Autodesk Fusion 360 part; units mm, degrees
note: some values were not read from the file. Set by a fixed rule: which face or edge a step refers to.
(part 3 of 3)
sketch "Sketch3" plane through (0, 0, 0) normal (0, -1, 0) x (1, 0, 0)
  line L0 (-40, 18) -> (-40, -18)
  line L1 (-40, -18) -> (40, -18)
  line L2 (40, -18) -> (40, 18)
  line L3 (40, 18) -> (-40, 18)
  line L4 (32.25, -8) -> (-32.25, -8)
  line L5 (-32.25, -8) -> (-32.25, 8)
  line L6 (-32.25, 8) -> (32.25, 8)
  line L7 (32.25, 8) -> (32.25, -8)
  line L8 (-40, 18) -> (40, -18) construction
  line L9 (-37, 15) -> (37, 15) construction
  line L10 (37, 15) -> (37, -15) construction
  line L11 (37, -15) -> (-37, -15) construction
  line L12 (-37, -15) -> (-37, 15) construction
  line L13 (-37, 15) -> (37, -15) construction
  line L14 (37, 15) -> (-37, -15) construction
  circle A0 centre (-37, 15) radius 2
  circle A1 centre (37, 15) radius 2
  circle A2 centre (-37, -15) radius 2
  circle A3 centre (37, -15) radius 2
  dimension "d13" = 74
  dimension "d14" = 4
  dimension "d15" = 4
  dimension "d16" = 4
  dimension "d17" = 4
  constraint coincident L0.start L3.end
  constraint coincident L1.end L2.start
  constraint horizontal L9
  constraint perpendicular L9 L10
  constraint parallel L9 L11
  constraint parallel L10 L12
  constraint coincident L13 origin
  constraint coincident L14 origin
  constraint coincident L9.start L12.end
  constraint coincident L9.end L10.start
  constraint coincident L11.end L12.start
  constraint coincident L10.end L11.start
  measures "d13" distance of L10.end L11.end
  measures "d14" diameter of A0
  measures "d15" diameter of A1
  measures "d16" diameter of A2
  measures "d17" diameter of A3
extrude "Extrude4" cut sketch "Sketch3" against normal blind 1.6 contours A0 | A1 | A2 | A3
fillet "Fillet1" radius 1 4 edges at (32.25, -3.2, 8) (32.25, -3.2, -8) (-32.25, -3.2, 8) (-32.25, -3.2, -8)
fillet "Fillet2" radius 0.5 8 edges at (-31.9571, -6.4, 7.7071) (-32.25, -6.4, 0) (-31.9571, -6.4, -7.7071) (0, -6.4, -8) (31.9571, -6.4, -7.7071) (32.25, -6.4, 0) (31.9571, -6.4, 7.7071) (0, -6.4, 8)
sketch "Sketch4" plane through (0, 0, 0) normal (0, -1, 0) x (1, 0, 0)
  line L0 (31.25, -8) -> (-31.25, -8)
  arc A0 (-32.25, -7) -> (-31.25, -8) centre (-31.25, -7) ccw
  line L1 (-32.25, -7) -> (-32.25, 7)
  arc A1 (-31.25, 8) -> (-32.25, 7) centre (-31.25, 7) ccw
  line L2 (-31.25, 8) -> (31.25, 8)
  arc A2 (32.25, 7) -> (31.25, 8) centre (31.25, 7) ccw
  line L3 (32.25, 7) -> (32.25, -7)
  arc A3 (31.25, -8) -> (32.25, -7) centre (31.25, -7) ccw
  line L4 (-40, 18) -> (-40, -18)
  line L5 (-40, -18) -> (40, -18)
  line L6 (40, -18) -> (40, 18)
  line L7 (40, 18) -> (-40, 18)
  circle A4 centre (37, 15) radius 2
  circle A5 centre (-37, 15) radius 2
  circle A6 centre (37, -15) radius 2
  circle A7 centre (-37, -15) radius 2
  line L8 (-30, 15) -> (-29.5, 15)
  line L9 (-29.5, 15) -> (-29.5, 15.5)
  line L10 (-29.5, 15.5) -> (-30, 15.5)
  line L11 (-30, 15.5) -> (-30, 15)
  dimension "d24" = 0.5
  dimension "d25" = 0.5
  constraint horizontal L8
  constraint vertical L9
  constraint horizontal L10
  constraint vertical L11
  measures "d24" distance of L8.start L8.end
  measures "d25" distance of L8.start L10.end
extrude "Extrude5" add sketch "Sketch4" along normal blind 2 contours L8 L9 L10 L11
fillet "Fillet3" radius 0.5 4 edges at (-29.75, 0, 15.5) (-29.5, 0, 15.25) (-29.75, 0, 15) (-30, 0, 15.25)
fillet "Fillet4" radius 0.1 4 edges at (-29.75, -2, 15.5) (-29.5, -2, 15.25) (-29.75, -2, 15) (-30, -2, 15.25)
pattern_linear "R-Pattern1" count 1 spacing 0 along (0, 0, -1) count 16 spacing 1.6667 along (1, 0, 0) of "Extrude5", "Fillet3", "Fillet4"
fillet "Fillet5" radius 0.5 4 edges at (40, 0.8, 18) (40, 0.8, -18) (-40, 0.8, 18) (-40, 0.8, -18)

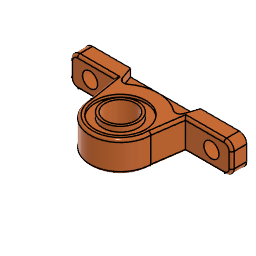
design "PillowBlock"
part number: 2026-09-24-15-42-36-700
Autodesk Fusion 360 part; units mm, degrees
sketch "Sketch1" plane through (0, 0, 0) normal (0, 0, 1) x (1, 0, 0)
  circle A0 centre (0, 0) radius 3
  line L0 (21, 21) -> (-21, 21) construction
  line L1 (-21, 21) -> (-21, -21) construction
  line L2 (-21, -21) -> (21, -21) construction
  line L3 (21, -21) -> (21, 21) construction
  line L4 (21, 21) -> (-21, -21) construction
  line L5 (-21, 21) -> (21, -21) construction
  circle A1 centre (0, 0) radius 6
  line L6 (21, 3) -> (-21, 3)
  line L7 (-21, 3) -> (-21, 9)
  line L8 (-21, 9) -> (21, 9)
  line L9 (21, 9) -> (21, 3)
  line L10 (21, 3) -> (-21, 9) construction
  line L11 (-21, 3) -> (21, 9) construction
  line L12 (0, 6) -> (21, 6)
  line L13 (0, 6) -> (-21, 6)
  line L14 (-6, -0.0008) -> (-6.9902, 6)
  line L15 (6, -0.0004) -> (6.8571, 5.9993)
  line L16 (6.4285, 2.9995) -> (6.8571, 5.9993)
  line L17 (6.4285, 2.9995) -> (6, -0.0004)
  line L18 (6.8571, 5.9993) -> (0, 6)
  point P0 (0, 6)
  dimension "d1" = 6
  dimension "d2" = 42
  dimension "d3" = 42
  dimension "d4" = 12
  dimension "d5" = 162.5
  constraint coincident A0.centre A1.centre
  constraint horizontal L0
  constraint perpendicular L0 L1
  constraint parallel L0 L2
  constraint parallel L1 L3
  constraint coincident L4 A0.centre
  constraint coincident L5 A0.centre
  constraint horizontal L6
  constraint perpendicular L6 L7
  constraint parallel L6 L8
  constraint parallel L7 L9
  constraint coincident L10 P0
  constraint coincident L11 P0
  constraint coincident L3 L6.start
  constraint coincident A1 P0
  constraint coincident P0 L12.start
  constraint midpoint L9 L12.end
  constraint midpoint L7 L13.end
  constraint coincident A1 L14.start
  constraint coincident L13 L14.end
  constraint coincident A1 L15.start
  constraint perpendicular L10 L15
  constraint midpoint L15 L16.start
  measures "d1" diameter of A0
  measures "d2" distance of L1.end L2.end
  measures "d3" distance of L0.end L1.end
  measures "d4" diameter of A1
  measures "d5" angle of L14 L15
extrude "Extrude1" add sketch "Sketch1" along normal blind 12 contours A1 L6 | A1 L6 | A1 L6 L15 L17 | A1 L6 L13 L14 | A1 L6 L14 | L7 L8 L9 L12 L13 L18
sketch "Sketch2" plane through (0, 0, 12) normal (0, 0, 1) x (-1, 0, 0)
  circle A0 centre (0, 0) radius 3
  arc A1 (6, 0.0008) -> (-6, 0.0004) centre (0, 0) ccw
  line L0 (-6, 0.0004) -> (-6.4286, -3)
  line L1 (-6.4286, -3) -> (-5.1962, -3)
  arc A2 (-5.1962, -3) -> (0, -6) centre (0, 0) ccw
  line L2 (0, -6) -> (-21, -6)
  line L3 (-21, -6) -> (-21, -9)
  line L4 (-21, -9) -> (21, -9)
  line L5 (21, -9) -> (21, -6)
  line L6 (21, -6) -> (6.9902, -6)
  line L7 (6.9902, -6) -> (6, 0.0008)
  line L8 (-6.2143, -1.4998) -> (-6.8572, -6)
  constraint midpoint L0 L8.start
  constraint coincident L2 L8.end
  constraint parallel L0 L8
extrude "Extrude2" add sketch "Sketch2" against normal blind 12 contours L1 A2 L2 L8
sketch "Sketch3" plane through (0, 0, 0) normal (0, 0, -1) x (1, 0, 0)
  circle A0 centre (0, 0) radius 3
  arc A1 (6, 0.0004) -> (-6, 0.0008) centre (0, 0) ccw
  line L0 (-6, 0.0008) -> (-6.9902, -6)
  line L1 (-6.9902, -6) -> (-21, -6)
  line L2 (-21, -6) -> (-21, -9)
  line L3 (-21, -9) -> (21, -9)
  line L4 (21, -9) -> (21, -6)
  line L5 (21, -6) -> (6.8572, -6)
  line L6 (6.8572, -6) -> (6, 0.0004)
  circle A2 centre (0, 0) radius 5
  dimension "d10" = 10
  constraint coincident A0.centre A1.centre
  measures "d10" diameter of A2
extrude "Extrude3" cut sketch "Sketch3" against normal blind 0.5 contours A2
sketch "Sketch4" plane through (0, 0, 0) normal (0, 0, -1) x (1, 0, 0)
  circle A0 centre (0, 0) radius 5
  arc A1 (6, 0.0004) -> (-6, 0.0008) centre (0, 0) ccw
  line L0 (-6, 0.0008) -> (-6.9902, -6)
  line L1 (-6.9902, -6) -> (-21, -6)
  line L2 (-21, -6) -> (-21, -9)
  line L3 (-21, -9) -> (21, -9)
  line L4 (21, -9) -> (21, -6)
  line L5 (21, -6) -> (6.8572, -6)
  line L6 (6.8572, -6) -> (6, 0.0004)
  line L7 (-6.9902, -9) -> (-6.9902, -6)
  line L8 (6.8572, -6) -> (6.8572, -9)
  line L9 (-4.8731, -4.9988) -> (4.8504, -4.9988)
  circle A2 centre (0, 0) radius 7.4924
  line L10 (5.8031, -5.6949) -> (6.8572, -9)
  line L11 (-5.8163, -5.6666) -> (-6.9902, -9)
  arc A3 (-4.8731, -4.9988) -> (-5.8163, -5.6666) centre (-4.8731, -5.9988) ccw
  arc A4 (5.8031, -5.6949) -> (4.8504, -4.9988) centre (4.8504, -5.9988) ccw
  dimension "d13" = 1
  constraint coincident L3 L7.start
  constraint coincident L0.end L1.start
  constraint perpendicular L1 L7
  constraint coincident L5.end L6.start
  constraint coincident L3 L8.end
  constraint perpendicular L3 L8
  constraint perpendicular L7 L9
  constraint coincident A0.centre A1.centre
  constraint tangent L11 A3
  constraint tangent L9 A3
  constraint tangent L10 A4
  constraint tangent L9 A4
  constraint equal A3 A4
  measures "d13" radius of A3
extrude "Extrude4" cut sketch "Sketch4" against normal blind 12 contours L3 A2 L10 L11 A3 A4
fillet "Fillet1" radius 1 2 edges at (-5.4267, 5.166, 6) (5.4178, 5.1753, 6)
sketch "Sketch5" plane through (0, 9, 0) normal (0, 1, 0) x (-1, 0, 0)
  line L0 (6.9902, 12) -> (6.9902, 0)
  line L1 (6.9902, 0) -> (21, 0)
  line L2 (21, 0) -> (21, 12)
  line L3 (21, 12) -> (6.9902, 12)
  line L4 (-21, 12) -> (21, 0) construction
  line L5 (21, 3) -> (-21, 3)
  line L6 (-21, 3) -> (-21, 9)
  line L7 (-21, 9) -> (21, 9)
  line L8 (21, 9) -> (21, 3)
  line L9 (21, 3) -> (-21, 9) construction
  line L10 (-21, 3) -> (21, 9) construction
  point P0 (0, 6)
  dimension "d18" = 6
  constraint coincident L1.end L2.start
  constraint horizontal L5
  constraint perpendicular L5 L6
  constraint parallel L5 L7
  constraint parallel L6 L8
  constraint coincident L9 P0
  constraint coincident L10 P0
  constraint midpoint L4 P0
  measures "d18" distance of L5.end L6.end
extrude "Extrude5" add sketch "Sketch5" against normal blind 3 contours L0 L2 L5 L7 L8 | L0 L5 L6 L7
sketch "Sketch6" plane through (0, 0, 12) normal (0, 0, 1) x (-1, 0, 0)
  line L0 (-6.8572, -9) -> (-6.0551, -6.4849)
  arc A0 (-4.5015, -5.9894) -> (-6.0551, -6.4849) centre (-5.1024, -6.7888) ccw
  arc A1 (-4.5015, -5.9894) -> (4.5356, -5.9636) centre (0, 0) ccw
  arc A2 (6.0842, -6.4274) -> (4.5356, -5.9636) centre (5.141, -6.7596) ccw
  line L1 (6.0842, -6.4274) -> (6.9902, -9)
  line L2 (6.9902, -9) -> (21, -9)
  line L3 (21, -9) -> (21, -6)
  line L4 (21, -6) -> (6.9902, -6)
  line L5 (6.9902, -6) -> (6, 0.0008)
  arc A3 (6, 0.0008) -> (-6, 0.0004) centre (0, 0) ccw
  line L6 (-6, 0.0004) -> (-6.8572, -6)
  line L7 (-6.8572, -6) -> (-21, -6)
  line L8 (-21, -6) -> (-21, -9)
  line L9 (-21, -9) -> (-6.8572, -9)
  circle A4 centre (0, 0) radius 3
  circle A5 centre (0, 0) radius 5
  dimension "d21" = 10
  constraint concentric A1 A5
  measures "d21" diameter of A5
extrude "Extrude6" cut sketch "Sketch6" against normal blind 0.5 contours A5
sketch "Sketch7" plane through (0, 0, 0.5) normal (0, 0, -1) x (1, 0, 0)
  circle A0 centre (0, 0) radius 3
  circle A1 centre (0, 0) radius 5
  circle A2 centre (0, 0) radius 3.5
  dimension "d24" = 7
  constraint coincident A0.centre A1.centre
  measures "d24" diameter of A2
extrude "Extrude7" add sketch "Sketch7" along normal blind 1 contours A2
extrude "Extrude8" add 1 faces at (3.3203, 0.1739, -0.5) along direction (0, 0, 1) blind 13
extrude "Extrude9" cut 1 faces at (11.5714, 6.9998, 12) along direction (0, 0, -1) blind 6
extrude "Extrude10" cut 1 faces at (-4.4814, 0.2484, 11.5) along direction (0, 0, -1) blind 6
extrude "Extrude11" cut 1 faces at (3.3203, 0.1739, 12.5) along direction (0, 0, -1) blind 6
extrude "Extrude12" cut 1 faces at (0.1337, 8.4911, 9) along direction (0, 0, -1) blind 6
sketch "Sketch8" plane through (0, 9, 0) normal (0, 1, 0) x (-1, 0, 0)
  line L0 (-6.8572, 0) -> (-6.8572, 6)
  line L1 (-6.8572, 6) -> (-21, 6)
  line L2 (-21, 6) -> (-21, 0)
  line L3 (-21, 0) -> (-6.8572, 0)
  line L4 (21, 0) -> (-21, 6) construction
  line L5 (-21, 4.5) -> (21, 4.5)
  line L6 (21, 4.5) -> (21, 1.5)
  line L7 (21, 1.5) -> (-21, 1.5)
  line L8 (-21, 1.5) -> (-21, 4.5)
  line L9 (-21, 4.5) -> (21, 1.5) construction
  line L10 (21, 4.5) -> (-21, 1.5) construction
  point P0 (0, 3)
  dimension "d37" = 3
  constraint coincident L1.end L2.start
  constraint horizontal L5
  constraint perpendicular L5 L6
  constraint parallel L5 L7
  constraint parallel L6 L8
  constraint coincident L9 P0
  constraint coincident L10 P0
  constraint midpoint L4 P0
  measures "d37" distance of L5.end L6.end
extrude "Extrude13" add sketch "Sketch8" against normal blind 3 contours L0 L2 L5 L7 L8 | L0 L5 L6 L7
extrude "Extrude14" cut 4 faces at (-21, 7, 0.5) (-21, 8, 5.5) (-21, 7, 2) (-21, 7, 3.5) along direction (1, 0, 0) blind 5
extrude "Extrude15" cut 4 faces at (21, 7, 2.5) (21, 8, 0.5) (21, 8, 3.5) (21, 7, 5.5) along direction (-1, 0, 0) blind 5
fillet "Fillet2" radius 1.5 4 edges at (-16, 7.5, 6) (-16, 7.5, 0) (16, 7.5, 0) (16, 7.5, 6)
sketch "Sketch9" plane through (0, 6, 0) normal (0, -1, 0) x (1, 0, 0)
  arc A0 (16, 4.5) -> (14.5, 6) centre (14.5, 4.5) ccw
  line L0 (14.5, 6) -> (6.8572, 6)
  line L1 (6.8572, 6) -> (6.8572, 0)
  line L2 (6.8572, 0) -> (14.5, 0)
  arc A1 (14.5, 0) -> (16, 1.5) centre (14.5, 1.5) ccw
  line L3 (16, 1.5) -> (16, 4.5)
  line L4 (16, 3) -> (12, 3) construction
  circle A2 centre (12, 3) radius 1.5
  dimension "d46" = 4
  dimension "d47" = 3
  constraint midpoint L3 L4.start
  constraint perpendicular L3 L4
  constraint coincident L4.end A2.centre
  measures "d46" distance of L4.start L4.end
  measures "d47" diameter of A2
extrude "Extrude16" cut sketch "Sketch9" against normal blind 3 contours A2
sketch "Sketch10" plane through (0, 6, 0) normal (0, -1, 0) x (1, 0, 0)
  arc A0 (-16, 1.5) -> (-14.5, 0) centre (-14.5, 1.5) ccw
  line L0 (-14.5, 0) -> (-6.9902, 0)
  line L1 (-6.9902, 0) -> (-6.9902, 6)
  line L2 (-6.9902, 6) -> (-14.5, 6)
  arc A1 (-14.5, 6) -> (-16, 4.5) centre (-14.5, 4.5) ccw
  line L3 (-16, 4.5) -> (-16, 1.5)
  line L4 (-16, 3) -> (-12, 3) construction
  circle A2 centre (-12, 3) radius 1.5
  dimension "d50" = 4
  dimension "d51" = 3
  constraint midpoint L3 L4.start
  constraint perpendicular L3 L4
  constraint coincident L4.end A2.centre
  measures "d50" distance of L4.start L4.end
  measures "d51" diameter of A2
extrude "Extrude17" cut sketch "Sketch10" against normal blind 3 contours A2
fillet "Fillet3" radius 0.5 16 edges at (0.0002, -6, 6) (-6.4951, 2.9996, 6) (6.4286, 2.9998, 6) (10.6786, 6, 0) (15.5607, 6, 0.4393) (16, 6, 3) (15.5607, 6, 5.5607) (10.6786, 6, 6) (-10.7451, 6, 6) (-15.5607, 6, 5.5607) (-16, 6, 3) (-15.5607, 6, 0.4393) (-10.7451, 6, 0) (-6.4951, 2.9996, 0) (0.0002, -6, 0) (6.4286, 2.9998, 0)

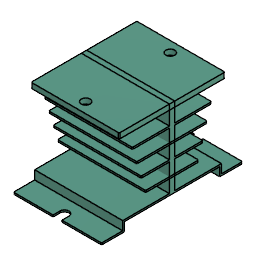
design "SSR_Heatsink"
part number: 2026-09-24-14-46-01-053
Autodesk Fusion 360 part; units mm, degrees
sketch "Sketch1" plane through (0, 0, 0) normal (0, 0, 1) x (1, 0, 0)
  line L0 (-25, 40) -> (25, 40) construction
  line L1 (25, 40) -> (25, -40) construction
  line L2 (25, -40) -> (-25, -40) construction
  line L3 (-25, -40) -> (-25, 40) construction
  line L4 (-25, 40) -> (25, -40) construction
  line L5 (25, 40) -> (-25, -40) construction
  line L6 (-25, 40) -> (25, 40)
  line L7 (25, 40) -> (25, 28)
  line L8 (25, 28) -> (-25, 28)
  line L9 (-25, 28) -> (-25, 40)
  line L10 (-25, -40) -> (25, -40)
  line L11 (25, -40) -> (25, -28)
  line L12 (25, -28) -> (-25, -28)
  line L13 (-25, -28) -> (-25, -40)
  dimension "d1" = 50
  dimension "d2" = 80
  dimension "d3" = 50
  dimension "d4" = 12
  dimension "d5" = 12
  constraint horizontal L0
  constraint perpendicular L0 L1
  constraint parallel L0 L2
  constraint parallel L1 L3
  constraint coincident L4 origin
  constraint coincident L5 origin
  constraint horizontal L6
  constraint vertical L7
  constraint horizontal L8
  constraint vertical L9
  constraint horizontal L10
  constraint vertical L11
  constraint horizontal L12
  constraint vertical L13
  measures "d1" distance of L1.end L2.end
  measures "d2" distance of L0.end L1.end
  measures "d3" distance of L0.start L0.end
  measures "d4" distance of L0.start L8.end
  measures "d5" distance of L2.end L12.end
extrude "Extrude1" add sketch "Sketch1" along normal blind 1 makes body 1 at (-8.3333, 36, 0) makes body 2 at (-8.3333, -32, 0)
sketch "Sketch2" plane through (0, 0, 0) normal (0, 0, 1) x (1, 0, 0)
  line L0 (-25, 40) -> (25, 40)
  line L1 (25, 40) -> (25, -40)
  line L2 (25, -40) -> (-25, -40)
  line L3 (-25, -40) -> (-25, 40)
  line L4 (-25, 40) -> (25, -40) construction
  line L5 (25, 40) -> (-25, -40) construction
  line L6 (-25, 28) -> (25, 28)
  line L7 (25, 28) -> (25, 27)
  line L8 (25, 27) -> (-25, 27)
  line L9 (-25, 27) -> (-25, 28)
  line L10 (-25, -28) -> (25, -28)
  line L11 (25, -28) -> (25, -27)
  line L12 (25, -27) -> (-25, -27)
  line L13 (-25, -27) -> (-25, -28)
  dimension "d8" = 1
  dimension "d9" = 1
  constraint horizontal L0
  constraint perpendicular L0 L1
  constraint parallel L0 L2
  constraint parallel L1 L3
  constraint coincident L4 origin
  constraint coincident L5 origin
  constraint horizontal L6
  constraint vertical L7
  constraint horizontal L8
  constraint vertical L9
  constraint coincident L3 L6.start
  constraint horizontal L10
  constraint vertical L11
  constraint horizontal L12
  constraint vertical L13
  constraint coincident L3 L10.start
  measures "d8" distance of L6.start L8.end
  measures "d9" distance of L10.start L12.end
extrude "Extrude2" add sketch "Sketch2" along normal blind 5 contours L1 L3 L6 L7 L8 L9 | L1 L3 L10 L11 L12 L13 bodies 1 2
ref_plane "WorkPlane1" through (0, -27.5, 5) normal (0, 0, 1) x (1, 0, 0)
sketch "Sketch3" plane through (0, 0, 5) normal (0, 0, 1) x (1, 0, 0)
  line L0 (-25, 28) -> (25, 28)
  line L1 (25, 28) -> (25, -28)
  line L2 (25, -28) -> (-25, -28)
  line L3 (-25, -28) -> (-25, 28)
  line L4 (-25, 28) -> (25, -28) construction
  line L5 (25, 28) -> (-25, -28) construction
  constraint horizontal L0
  constraint perpendicular L0 L1
  constraint parallel L0 L2
  constraint parallel L1 L3
  constraint coincident L4 origin
  constraint coincident L5 origin
extrude "Extrude3" add sketch "Sketch3" along normal blind 1 bodies 1 2
sketch "Sketch4" plane through (0, 0, 6) normal (0, 0, 1) x (-1, 0, 0)
  line L0 (25, 28) -> (-25, 28)
  line L1 (-25, 28) -> (-25, -28)
  line L2 (-25, -28) -> (25, -28)
  line L3 (25, -28) -> (25, 28)
  line L4 (-25, 15) -> (25, 15)
  line L5 (25, 15) -> (25, -15)
  line L6 (25, -15) -> (-25, -15)
  line L7 (-25, -15) -> (-25, 15)
  line L8 (-25, 15) -> (25, -15) construction
  line L9 (25, 15) -> (-25, -15) construction
  line L10 (25, 1.5) -> (-25, 1.5)
  line L11 (-25, 1.5) -> (-25, -1.5)
  line L12 (-25, -1.5) -> (25, -1.5)
  line L13 (25, -1.5) -> (25, 1.5)
  line L14 (25, 1.5) -> (-25, -1.5) construction
  line L15 (-25, 1.5) -> (25, -1.5) construction
  dimension "d15" = 30
  dimension "d16" = 3
  constraint horizontal L4
  constraint perpendicular L4 L5
  constraint parallel L4 L6
  constraint parallel L5 L7
  constraint coincident L8 origin
  constraint coincident L9 origin
  constraint horizontal L10
  constraint perpendicular L10 L11
  constraint parallel L10 L12
  constraint parallel L11 L13
  constraint coincident L14 origin
  constraint coincident L15 origin
  measures "d15" distance of L4.end L5.end
  measures "d16" distance of L10.end L11.end
extrude "Extrude4" add sketch "Sketch4" along normal blind 44 contours L1 L3 L5 L7 L10 L11 L12 L13 bodies 1
ref_plane "WorkPlane2" through (0, 14.75, 13.3) normal (0, 0, 1) x (1, 0, 0)
sketch "Sketch5" plane through (0, 0, 13.3) normal (0, 0, 1) x (1, 0, 0)
  line L0 (25, -15) -> (-25, -15)
  line L1 (-25, -15) -> (-25, 15)
  line L2 (-25, 15) -> (25, 15)
  line L3 (25, 15) -> (25, -15)
  line L4 (25, -15) -> (-25, 15) construction
  line L5 (-25, -15) -> (25, 15) construction
  constraint horizontal L0
  constraint perpendicular L0 L1
  constraint parallel L0 L2
  constraint parallel L1 L3
  constraint coincident L4 origin
  constraint coincident L5 origin
extrude "Extrude5" add sketch "Sketch5" along normal blind 1 separate body makes body 3
ref_plane "WorkPlane3" through (0, 0, 21.6) normal (0, 0, 1) x (1, 0, 0)
sketch "Sketch6" plane through (0, 0, 21.6) normal (0, 0, 1) x (1, 0, 0)
  line L0 (25, -17.5) -> (-25, -17.5)
  line L1 (-25, -17.5) -> (-25, 17.5)
  line L2 (-25, 17.5) -> (25, 17.5)
  line L3 (25, 17.5) -> (25, -17.5)
  line L4 (25, -17.5) -> (-25, 17.5) construction
  line L5 (-25, -17.5) -> (25, 17.5) construction
  dimension "d23" = 35
  constraint horizontal L0
  constraint perpendicular L0 L1
  constraint parallel L0 L2
  constraint parallel L1 L3
  constraint coincident L4 origin
  constraint coincident L5 origin
  measures "d23" distance of L0.end L1.end
extrude "Extrude6" add sketch "Sketch6" along normal blind 1 bodies 1
ref_plane "WorkPlane4" through (0, 9.5, 29.9) normal (0, 0, 1) x (1, 0, 0)
sketch "Sketch7" plane through (0, 0, 29.9) normal (0, 0, 1) x (1, 0, 0)
  line L0 (25, -20) -> (-25, -20)
  line L1 (-25, -20) -> (-25, 20)
  line L2 (-25, 20) -> (25, 20)
  line L3 (25, 20) -> (25, -20)
  line L4 (25, -20) -> (-25, 20) construction
  line L5 (-25, -20) -> (25, 20) construction
  dimension "d27" = 50
  dimension "d28" = 40
  constraint horizontal L0
  constraint perpendicular L0 L1
  constraint parallel L0 L2
  constraint parallel L1 L3
  constraint coincident L4 origin
  constraint coincident L5 origin
  measures "d27" distance of L1.end L2.end
  measures "d28" distance of L0.end L1.end
extrude "Extrude7" add sketch "Sketch7" along normal blind 1 separate body makes body 4
ref_plane "WorkPlane5" through (0, 0, 38.2) normal (0, 0, 1) x (1, 0, 0)
sketch "Sketch8" plane through (0, 0, 38.2) normal (0, 0, 1) x (1, 0, 0)
  line L0 (25, -22.5) -> (-25, -22.5)
  line L1 (-25, -22.5) -> (-25, 22.5)
  line L2 (-25, 22.5) -> (25, 22.5)
  line L3 (25, 22.5) -> (25, -22.5)
  line L4 (25, -22.5) -> (-25, 22.5) construction
  line L5 (-25, -22.5) -> (25, 22.5) construction
  dimension "d32" = 45
  constraint horizontal L0
  constraint perpendicular L0 L1
  constraint parallel L0 L2
  constraint parallel L1 L3
  constraint coincident L4 origin
  constraint coincident L5 origin
  measures "d32" distance of L0.end L1.end
extrude "Extrude8" add sketch "Sketch8" along normal blind 1 bodies 1
ref_plane "WorkPlane6" through (0, 0, 50) normal (0, 0, 1) x (1, 0, 0)
sketch "Sketch9" plane through (0, 0, 50) normal (0, 0, 1) x (1, 0, 0)
  line L0 (25, -30) -> (-25, -30)
  line L1 (-25, -30) -> (-25, 30)
  line L2 (-25, 30) -> (25, 30)
  line L3 (25, 30) -> (25, -30)
  line L4 (25, -30) -> (-25, 30) construction
  line L5 (-25, -30) -> (25, 30) construction
  dimension "d36" = 50
  dimension "d37" = 60
  constraint horizontal L0
  constraint perpendicular L0 L1
  constraint parallel L0 L2
  constraint parallel L1 L3
  constraint coincident L4 origin
  constraint coincident L5 origin
  measures "d36" distance of L1.end L2.end
  measures "d37" distance of L0.end L1.end
extrude "Extrude9" add sketch "Sketch9" against normal blind 3 separate body makes body 5
sketch "Sketch10" plane through (0, 0, 50) normal (0, 0, 1) x (-1, 0, 0)
  line L0 (-25, -30) -> (25, -30)
  line L1 (25, -30) -> (25, 30)
  line L2 (25, 30) -> (-25, 30)
  line L3 (-25, 30) -> (-25, -30)
  line L4 (-24, 24) -> (24, 24) construction
  line L5 (24, 24) -> (24, -24) construction
  line L6 (24, -24) -> (-24, -24) construction
  line L7 (-24, -24) -> (-24, 24) construction
  line L8 (-24, 24) -> (24, -24) construction
  line L9 (24, 24) -> (-24, -24) construction
  circle A0 centre (0, 24) radius 2.5
  circle A1 centre (0, -24) radius 2.5
  dimension "d40" = 48
  dimension "d41" = 48
  dimension "d42" = 5
  dimension "d43" = 5
  constraint horizontal L4
  constraint perpendicular L4 L5
  constraint parallel L4 L6
  constraint parallel L5 L7
  constraint coincident L8 origin
  constraint coincident L9 origin
  constraint midpoint L4 A0.centre
  constraint midpoint L6 A1.centre
  measures "d40" distance of L5.end L6.end
  measures "d41" distance of L4.end L5.end
  measures "d42" diameter of A0
  measures "d43" diameter of A1
extrude "Extrude10" cut sketch "Sketch10" against normal blind 3 contours A0 | A1 bodies 5
sketch "Sketch11" plane through (0, 0, 1) normal (0, 0, 1) x (-1, 0, 0)
  line L0 (25, -28) -> (-25, -28)
  line L1 (-25, -28) -> (-25, -40)
  line L2 (-25, -40) -> (25, -40)
  line L3 (25, -40) -> (25, -28)
  line L4 (2.5, -44) -> (2.5, -36)
  arc A0 (2.5, -36) -> (-2.5, -36) centre (0, -36) ccw
  line L5 (-2.5, -36) -> (-2.5, -44)
  arc A1 (-2.5, -44) -> (2.5, -44) centre (0, -44) ccw
  line L6 (0, -44) -> (0, -36) construction
  point P0 (0, -40)
  dimension "d46" = 5
  constraint tangent L4 A0
  constraint tangent A0 L5
  constraint parallel L4 L5
  constraint tangent L5 A1
  constraint tangent L4 A1
  constraint perpendicular L2 L6
  constraint midpoint L2 P0
  constraint midpoint L6 P0
  measures "d46" diameter of A0
extrude "Extrude11" cut sketch "Sketch11" against normal blind 1 contours L2 L4 A0 L5 bodies 1
sketch "Sketch12" plane through (0, 0, 1) normal (0, 0, 1) x (-1, 0, 0)
  line L0 (25, 28) -> (25, 40)
  line L1 (25, 40) -> (-25, 40)
  line L2 (-25, 40) -> (-25, 28)
  line L3 (-25, 28) -> (25, 28)
  line L4 (-2.5, 44) -> (-2.5, 36)
  arc A0 (-2.5, 36) -> (2.5, 36) centre (0, 36) ccw
  line L5 (2.5, 36) -> (2.5, 44)
  arc A1 (2.5, 44) -> (-2.5, 44) centre (0, 44) ccw
  line L6 (0, 44) -> (0, 36) construction
  point P0 (0, 40)
  dimension "d49" = 5
  constraint tangent L4 A0
  constraint tangent A0 L5
  constraint parallel L4 L5
  constraint tangent L5 A1
  constraint tangent L4 A1
  constraint perpendicular L1 L6
  constraint midpoint L1 P0
  constraint midpoint L6 P0
  measures "d49" diameter of A0
extrude "Extrude12" cut sketch "Sketch12" against normal blind 1 contours L1 L4 A0 L5 bodies 1
fillet "Fillet1" radius 0.5 23 edges at (25, -22.5, 38.7) (25, -17.5, 22.1) (25, -40, 0.5) (-25, -40, 0.5) (25, 40, 0.5) (25, 17.5, 22.1) (25, 22.5, 38.7) (-25, 40, 0.5) (-25, 17.5, 22.1) (-25, -22.5, 38.7) (-25, -17.5, 22.1) (25, -15, 13.8) (25, 15, 13.8) (-25, 15, 13.8) (-25, -15, 13.8) (25, -20, 30.4) (25, 20, 30.4) (-25, 20, 30.4) (-25, -20, 30.4) (25, -30, 48.5) (25, 30, 48.5) (-25, 30, 48.5) (-25, -30, 48.5) on bodies 1 3 4 5

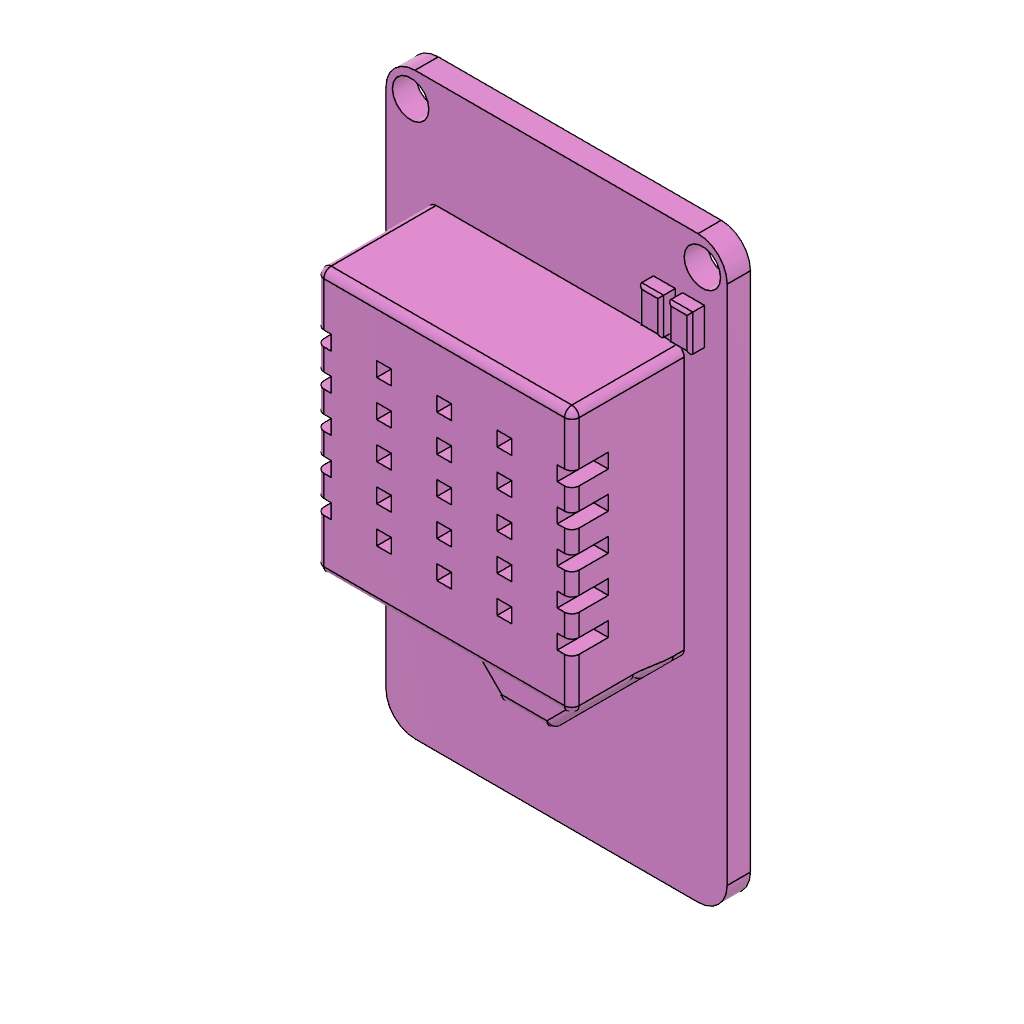
design "DHT22"
part number: 2026-09-25-09-54-51-033
Autodesk Fusion 360 part; units mm, degrees
sketch "Sketch1" plane through (0, 0, 0) normal (0, 0, 1) x (1, 0, 0)
  line L0 (-11.7, 19.85) -> (11.7, 19.85)
  line L1 (11.7, 19.85) -> (11.7, -19.85)
  line L2 (11.7, -19.85) -> (-11.7, -19.85)
  line L3 (-11.7, -19.85) -> (-11.7, 19.85)
  line L4 (-11.7, 19.85) -> (11.7, -19.85) construction
  line L5 (11.7, 19.85) -> (-11.7, -19.85) construction
  dimension "d1" = 23.4
  dimension "d2" = 39.7
  constraint horizontal L0
  constraint perpendicular L0 L1
  constraint parallel L0 L2
  constraint parallel L1 L3
  constraint coincident L4 origin
  constraint coincident L5 origin
  measures "d1" distance of L1.end L2.end
  measures "d2" distance of L0.end L1.end
extrude "Extrude1" add sketch "Sketch1" along normal blind 1.6
sketch "Sketch2" plane through (0, 0, 1.6) normal (0, 0, 1) x (1, 0, 0)
  line L0 (-11.7, -19.85) -> (11.7, -19.85)
  line L1 (11.7, -19.85) -> (11.7, 19.85)
  line L2 (11.7, 19.85) -> (-11.7, 19.85)
  line L3 (-11.7, 19.85) -> (-11.7, -19.85)
  line L4 (-8.75, 12.55) -> (8.75, 12.55)
  line L5 (8.75, 12.55) -> (8.75, -12.55)
  line L6 (8.75, -12.55) -> (-8.75, -12.55)
  line L7 (-8.75, -12.55) -> (-8.75, 12.55)
  line L8 (-8.75, 12.55) -> (8.75, -12.55) construction
  line L9 (8.75, 12.55) -> (-8.75, -12.55) construction
  dimension "d5" = 17.5
  dimension "d6" = 25.1
  constraint horizontal L4
  constraint perpendicular L4 L5
  constraint parallel L4 L6
  constraint parallel L5 L7
  constraint coincident L8 origin
  constraint coincident L9 origin
  measures "d5" distance of L5.end L6.end
  measures "d6" distance of L4.end L5.end
extrude "Extrude2" add sketch "Sketch2" along normal blind 7.7 contours L4 L5 L6 L7
sketch "Sketch3" plane through (0, 0, 9.3) normal (0, 0, 1) x (1, 0, 0)
  line L0 (-8.75, -12.55) -> (8.75, -12.55)
  line L1 (8.75, -12.55) -> (8.75, 12.55)
  line L2 (8.75, 12.55) -> (-8.75, 12.55)
  line L3 (-8.75, 12.55) -> (-8.75, -12.55)
  line L4 (-8.75, -12.55) -> (8.75, -12.55)
  line L5 (8.75, -12.55) -> (8.75, -5.55)
  line L6 (8.75, -5.55) -> (-8.75, -5.55)
  line L7 (-8.75, -5.55) -> (-8.75, -12.55)
  dimension "d9" = 7
  constraint horizontal L4
  constraint vertical L5
  constraint horizontal L6
  constraint vertical L7
  constraint coincident L0.start L3.end
  measures "d9" distance of L0.start L6.end
extrude "Extrude3" cut sketch "Sketch3" against normal blind 5.5 contours L0 L1 L3 L4 L5 L6 L7
chamfer "Chamfer1" distance 7 angle 45 2 edges at (8.75, -12.55, 2.7) (-8.75, -12.55, 2.7)
fillet "Fillet1" radius 0.5 12 edges at (1.75, -12.55, 2.7) (-1.75, -12.55, 2.7) (8.75, -5.55, 2.7) (-8.75, -5.55, 2.7) (-8.75, -5.55, 6.55) (8.75, -5.55, 6.55) (0, -5.55, 9.3) (8.75, 3.5, 9.3) (-8.75, 3.5, 9.3) (0, 12.55, 9.3) (8.75, 12.55, 5.45) (-8.75, 12.55, 5.45) 1 faces at (0.5833, -7.8833, 3.8)
sketch "Sketch4" plane through (0, 0, 3.8) normal (0, 0, 1) x (1, 0, 0)
  line L0 (-1.5429, -12.05) -> (1.5429, -12.05)
  line L1 (1.5429, -12.05) -> (7.2299, -6.363)
  arc A0 (7.2299, -6.363) -> (7.1003, -6.05) centre (7.1003, -6.2333) ccw
  line L2 (7.1003, -6.05) -> (-7.1003, -6.05)
  arc A1 (-7.1003, -6.05) -> (-7.2299, -6.363) centre (-7.1003, -6.2333) ccw
  line L3 (-7.2299, -6.363) -> (-1.5429, -12.05)
  line L4 (0, -6.05) -> (0, -12.05) construction
  circle A2 centre (0, -9.05) radius 1.5
  dimension "d15" = 3
  constraint midpoint L2 L4.start
  constraint midpoint L0 L4.end
  constraint midpoint L4 A2.centre
  measures "d15" diameter of A2
extrude "Extrude4" cut sketch "Sketch4" against normal blind 2.2 contours A2
sketch "Sketch5" plane through (0, 0, 9.3) normal (0, 0, 1) x (1, 0, 0)
  line L0 (8.25, 12.05) -> (-8.25, 12.05)
  line L1 (-8.25, 12.05) -> (-8.25, -5.05)
  line L2 (-8.25, -5.05) -> (8.25, -5.05)
  line L3 (8.25, -5.05) -> (8.25, 12.05)
  line L4 (-8.25, 12.05) -> (8.25, -5.05) construction
  line L5 (-0.5, 4) -> (0.5, 4)
  line L6 (0.5, 4) -> (0.5, 3)
  line L7 (0.5, 3) -> (-0.5, 3)
  line L8 (-0.5, 3) -> (-0.5, 4)
  line L9 (-0.5, 4) -> (0.5, 3) construction
  line L10 (0.5, 4) -> (-0.5, 3) construction
  point P0 (0, 3.5)
  dimension "d18" = 1
  dimension "d19" = 1
  constraint coincident L0.end L1.start
  constraint coincident L2.end L3.start
  constraint horizontal L5
  constraint perpendicular L5 L6
  constraint parallel L5 L7
  constraint parallel L6 L8
  constraint coincident L9 P0
  constraint coincident L10 P0
  constraint midpoint L4 P0
  measures "d18" distance of L6.end L7.end
  measures "d19" distance of L5.end L6.end
extrude "Extrude5" cut sketch "Sketch5" against normal blind 2.5 contours L5 L6 L7 L8
pattern_linear "R-Pattern1" count 5 spacing 2.5 along (0, -1, 0) both ways count 5 spacing 4.125 along (-1, 0, 0) both ways of "Extrude5"
sketch "Sketch6" plane through (0, 0, 1.6) normal (0, 0, 1) x (1, 0, 0)
  line L0 (-8.75, -5.3429) -> (-8.75, 12.05)
  arc A0 (-8.25, 12.55) -> (-8.75, 12.05) centre (-8.25, 12.05) ccw
  line L1 (-8.25, 12.55) -> (8.25, 12.55)
  arc A1 (8.75, 12.05) -> (8.25, 12.55) centre (8.25, 12.05) ccw
  line L2 (8.75, 12.05) -> (8.75, -5.3429)
  arc A2 (8.6036, -5.6964) -> (8.75, -5.3429) centre (8.25, -5.3429) ccw
  line L3 (8.6036, -5.6964) -> (1.8964, -12.4036)
  arc A3 (1.5429, -12.55) -> (1.8964, -12.4036) centre (1.5429, -12.05) ccw
  line L4 (1.5429, -12.55) -> (-1.5429, -12.55)
  arc A4 (-1.8964, -12.4036) -> (-1.5429, -12.55) centre (-1.5429, -12.05) ccw
  line L5 (-1.8964, -12.4036) -> (-8.6036, -5.6964)
  arc A5 (-8.75, -5.3429) -> (-8.6036, -5.6964) centre (-8.25, -5.3429) ccw
  line L6 (-11.7, -19.85) -> (11.7, -19.85)
  line L7 (11.7, -19.85) -> (11.7, 19.85)
  line L8 (11.7, 19.85) -> (-11.7, 19.85)
  line L9 (-11.7, 19.85) -> (-11.7, -19.85)
  line L10 (10, -18) -> (-10, -18) construction
  line L11 (-10, -18) -> (-10, 18) construction
  line L12 (-10, 18) -> (10, 18) construction
  line L13 (10, 18) -> (10, -18) construction
  line L14 (10, -18) -> (-10, 18) construction
  line L15 (-10, -18) -> (10, 18) construction
  circle A6 centre (-10, 18) radius 1.25
  circle A7 centre (10, 18) radius 1.25
  dimension "d26" = 20
  dimension "d27" = 36
  dimension "d28" = 2.5
  dimension "d29" = 2.5
  constraint horizontal L10
  constraint perpendicular L10 L11
  constraint parallel L10 L12
  constraint parallel L11 L13
  constraint coincident L14 origin
  constraint coincident L15 origin
  constraint coincident L11.end L12.start
  constraint coincident L12.end L13.start
  measures "d26" distance of L11.end L12.end
  measures "d27" distance of L10.end L11.end
  measures "d28" diameter of A6
  measures "d29" diameter of A7
extrude "Extrude6" cut sketch "Sketch6" against normal blind 1.6 contours A6 | A7
fillet "Fillet2" radius 2 4 edges at (11.7, 19.85, 0.8) (-11.7, 19.85, 0.8) (11.7, -19.85, 0.8) (-11.7, -19.85, 0.8)
sketch "Sketch7" plane through (0, 0, 1.6) normal (0, 0, 1) x (1, 0, 0)
  arc A0 (-11.7, -17.85) -> (-9.7, -19.85) centre (-9.7, -17.85) ccw
  line L0 (-9.7, -19.85) -> (9.7, -19.85)
  arc A1 (9.7, -19.85) -> (11.7, -17.85) centre (9.7, -17.85) ccw
  line L1 (11.7, -17.85) -> (11.7, 17.85)
  arc A2 (11.7, 17.85) -> (9.7, 19.85) centre (9.7, 17.85) ccw
  line L2 (9.7, 19.85) -> (-9.7, 19.85)
  arc A3 (-9.7, 19.85) -> (-11.7, 17.85) centre (-9.7, 17.85) ccw
  line L3 (-11.7, 17.85) -> (-11.7, -17.85)
  circle A4 centre (10, 18) radius 1.25
  circle A5 centre (-10, 18) radius 1.25
  line L4 (-8.75, -5.3429) -> (-8.75, 12.05)
  arc A6 (-8.25, 12.55) -> (-8.75, 12.05) centre (-8.25, 12.05) ccw
  line L5 (-8.25, 12.55) -> (8.25, 12.55)
  arc A7 (8.75, 12.05) -> (8.25, 12.55) centre (8.25, 12.05) ccw
  line L6 (8.75, 12.05) -> (8.75, -5.3429)
  arc A8 (8.6036, -5.6964) -> (8.75, -5.3429) centre (8.25, -5.3429) ccw
  line L7 (8.6036, -5.6964) -> (1.8964, -12.4036)
  arc A9 (1.5429, -12.55) -> (1.8964, -12.4036) centre (1.5429, -12.05) ccw
  line L8 (1.5429, -12.55) -> (-1.5429, -12.55)
  arc A10 (-1.8964, -12.4036) -> (-1.5429, -12.55) centre (-1.5429, -12.05) ccw
  line L9 (-1.8964, -12.4036) -> (-8.6036, -5.6964)
  arc A11 (-8.75, -5.3429) -> (-8.6036, -5.6964) centre (-8.25, -5.3429) ccw
  line L10 (10.1435, 13.315) -> (8.6435, 13.315)
  line L11 (8.6435, 13.315) -> (8.6435, 15.815)
  line L12 (8.6435, 15.815) -> (10.1435, 15.815)
  line L13 (10.1435, 15.815) -> (10.1435, 13.315)
  dimension "d34" = 1.5
  dimension "d35" = 2.5
  constraint horizontal L10
  constraint vertical L11
  constraint horizontal L12
  constraint vertical L13
  measures "d34" distance of L10.start L10.end
  measures "d35" distance of L10.start L12.end
extrude "Extrude7" add sketch "Sketch7" along normal blind 1 contours L10 L11 L12 L13
pattern_linear "R-Pattern2" count 1 spacing 0 along (0, -1, 0) count 2 spacing 2 along (-1, 0, 0) of "Extrude7"
fillet "Fillet3" radius 0.2 2 faces at (9.6435, 14.1484, 2.6) (7.6435, 14.1484, 2.6)

design "PTCHeater"
part number: 2026-09-24-10-30-13-684
Autodesk Fusion 360 part; units mm, degrees
sketch "Sketch1" plane through (0, 0, 0) normal (0, 0, 1) x (1, 0, 0)
  line L0 (9.5, 30) -> (-9.5, 30)
  line L1 (-9.5, 30) -> (-9.5, -30)
  line L2 (-9.5, -30) -> (9.5, -30)
  line L3 (9.5, -30) -> (9.5, 30)
  line L4 (9.5, 30) -> (-9.5, -30) construction
  line L5 (-9.5, 30) -> (9.5, -30) construction
  line L6 (-9.5, -30) -> (9.5, -30)
  line L7 (9.5, -30) -> (9.5, -29.5)
  line L8 (9.5, -29.5) -> (-9.5, -29.5)
  line L9 (-9.5, -29.5) -> (-9.5, -30)
  line L10 (9.5, -29.5) -> (9, -29.5)
  line L11 (9, -29.5) -> (9, -29)
  line L12 (9, -29) -> (9.5, -29)
  line L13 (9.5, -29) -> (9.5, -29.5)
  line L14 (9.5, -29) -> (-9.5, -29)
  line L15 (-9.5, -29) -> (-9.5, -28.5)
  line L16 (-9.5, -28.5) -> (9.5, -28.5)
  line L17 (9.5, -28.5) -> (9.5, -29)
  line L18 (-9.5, -28.5) -> (-9, -28.5)
  line L19 (-9, -28.5) -> (-9, -28)
  line L20 (-9, -28) -> (-9.5, -28)
  line L21 (-9.5, -28) -> (-9.5, -28.5)
  dimension "d1" = 19
  dimension "d2" = 60
  dimension "d3" = 0.5
  dimension "d4" = 0.5
  dimension "d5" = 0.5
  dimension "d6" = 0.5
  dimension "d7" = 0.5
  dimension "d8" = 0.5
  constraint horizontal L0
  constraint perpendicular L0 L1
  constraint parallel L0 L2
  constraint parallel L1 L3
  constraint coincident L4 origin
  constraint coincident L5 origin
  constraint horizontal L6
  constraint vertical L7
  constraint horizontal L8
  constraint vertical L9
  constraint horizontal L10
  constraint vertical L11
  constraint horizontal L12
  constraint vertical L13
  constraint horizontal L14
  constraint vertical L15
  constraint horizontal L16
  constraint vertical L17
  constraint horizontal L18
  constraint vertical L19
  constraint horizontal L20
  constraint vertical L21
  measures "d1" distance of L1.end L2.end
  measures "d2" distance of L0.end L1.end
  measures "d3" distance of L1.end L8.end
  measures "d4" distance of L7.end L10.end
  measures "d5" distance of L7.end L12.end
  measures "d6" distance of L12.end L16.end
  measures "d7" distance of L15.end L18.end
  measures "d8" distance of L15.end L20.end
extrude "Extrude1" add sketch "Sketch1" along normal blind 20 contours L1 L3 L12 L14 L15 L16 L17 L18 | L1 L16 L18 L19 L20 L21 | L3 L8 L10 L11 L12 L13 L14 | L1 L2 L3 L6 L7 L8 L9 L10 makes body 1
fillet "Fillet1" radius 0.75 4 edges at (9.5, -28.5, 10) (9.5, -30, 10) (-9.5, -29, 10) (-9.5, -29.5, 10) on bodies 1
pattern_linear "R-Pattern1" count 1 spacing 0 along (-1, 0, 0) count 30 spacing 2 along (0, 1, 0) of "Extrude1", "Fillet1" makes body 2 at (-3.4167, -28, 6.6667) makes body 3 at (-3.4167, -26, 6.6667) makes body 4 at (-3.4167, -24, 6.6667) makes body 5 at (-3.4167, -22, 6.6667) makes body 6 at (-3.4167, -20, 6.6667) makes body 7 at (-3.4167, -18, 6.6667) makes body 8 at (-3.4167, -16, 6.6667) makes body 9 at (-3.4167, -14, 6.6667) makes body 10 at (-3.4167, -12, 6.6667) makes body 11 at (-3.4167, -10, 6.6667) makes body 12 at (-3.4167, -8, 6.6667) makes body 13 at (-3.4167, -6, 6.6667) makes body 14 at (-3.4167, -4, 6.6667) makes body 15 at (-3.4167, -2, 6.6667) makes body 16 at (-3.4167, 0, 6.6667) makes body 17 at (-3.4167, 2, 6.6667) makes body 18 at (-3.4167, 4, 6.6667) makes body 19 at (-3.4167, 6, 6.6667) makes body 20 at (-3.4167, 8, 6.6667) makes body 21 at (-3.4167, 10, 6.6667) makes body 22 at (-3.4167, 12, 6.6667) makes body 23 at (-3.4167, 14, 6.6667) makes body 24 at (-3.4167, 16, 6.6667) makes body 25 at (-3.4167, 18, 6.6667) makes body 26 at (-3.4167, 20, 6.6667) makes body 27 at (-3.4167, 22, 6.6667) makes body 28 at (-3.4167, 24, 6.6667) makes body 29 at (-3.4167, 26, 6.6667) makes body 30 at (-3.4167, 28, 6.6667)
pattern_linear "R-Pattern2" count 1 spacing 0 along (0, 1, 0) count 3 spacing 20 along (1, 0, 0) of "Extrude1", "Fillet1", "R-Pattern1" makes body 31 at (16.5833, -30, 6.6667) makes body 32 at (36.5833, -30, 6.6667) makes body 33 at (16.5833, -28, 6.6667) makes body 34 at (36.5833, -28, 6.6667) makes body 35 at (16.5833, -26, 6.6667) makes body 36 at (36.5833, -26, 6.6667) makes body 37 at (16.5833, -24, 6.6667) makes body 38 at (36.5833, -24, 6.6667) makes body 39 at (16.5833, -22, 6.6667) makes body 40 at (36.5833, -22, 6.6667) makes body 41 at (16.5833, -20, 6.6667) makes body 42 at (36.5833, -20, 6.6667) makes body 43 at (16.5833, -18, 6.6667) makes body 44 at (36.5833, -18, 6.6667) makes body 45 at (16.5833, -16, 6.6667) makes body 46 at (36.5833, -16, 6.6667) makes body 47 at (16.5833, -14, 6.6667) makes body 48 at (36.5833, -14, 6.6667) makes body 49 at (16.5833, -12, 6.6667) makes body 50 at (36.5833, -12, 6.6667) makes body 51 at (16.5833, -10, 6.6667) makes body 52 at (36.5833, -10, 6.6667) makes body 53 at (16.5833, -8, 6.6667) makes body 54 at (36.5833, -8, 6.6667) makes body 55 at (16.5833, -6, 6.6667) makes body 56 at (36.5833, -6, 6.6667) makes body 57 at (16.5833, -4, 6.6667) makes body 58 at (36.5833, -4, 6.6667) makes body 59 at (16.5833, -2, 6.6667) makes body 60 at (36.5833, -2, 6.6667) makes body 61 at (16.5833, 0, 6.6667) makes body 62 at (36.5833, 0, 6.6667) makes body 63 at (16.5833, 2, 6.6667) makes body 64 at (36.5833, 2, 6.6667) makes body 65 at (16.5833, 4, 6.6667) makes body 66 at (36.5833, 4, 6.6667) makes body 67 at (16.5833, 6, 6.6667) makes body 68 at (36.5833, 6, 6.6667) makes body 69 at (16.5833, 8, 6.6667) makes body 70 at (36.5833, 8, 6.6667) makes body 71 at (16.5833, 10, 6.6667) makes body 72 at (36.5833, 10, 6.6667) makes body 73 at (16.5833, 12, 6.6667) makes body 74 at (36.5833, 12, 6.6667) makes body 75 at (16.5833, 14, 6.6667) makes body 76 at (36.5833, 14, 6.6667) makes body 77 at (16.5833, 16, 6.6667) makes body 78 at (36.5833, 16, 6.6667) makes body 79 at (16.5833, 18, 6.6667) makes body 80 at (36.5833, 18, 6.6667) makes body 81 at (16.5833, 20, 6.6667) makes body 82 at (36.5833, 20, 6.6667) makes body 83 at (16.5833, 22, 6.6667) makes body 84 at (36.5833, 22, 6.6667) makes body 85 at (16.5833, 24, 6.6667) makes body 86 at (36.5833, 24, 6.6667) makes body 87 at (16.5833, 26, 6.6667) makes body 88 at (36.5833, 26, 6.6667) makes body 89 at (16.5833, 28, 6.6667) makes body 90 at (36.5833, 28, 6.6667)
